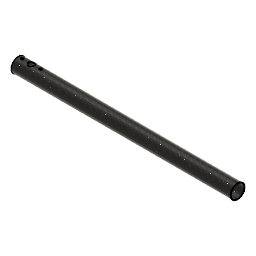
onlydrone (Autodesk Fusion 360 archive; units mm, degrees)
design "Arm"
Autodesk Fusion 360 part; units mm, degrees
sketch "Sketch1" plane through (0, 0, 0) normal (1, 0, 0) x (0, 1, 0)
  circle A0 centre (0, 0) radius 10
  circle A1 centre (0, 0) radius 9
  dimension "d1" = 20
  dimension "d2" = 18
  constraint coincident A0.centre A1.centre
  measures "d1" diameter of A0
  measures "d2" diameter of A1
extrude "Extrude1" add sketch "Sketch1" along normal blind 300
sketch "Sketch2" plane through (0, 0, 0) normal (0, 0, 1) x (1, 0, 0)
  line L0 (0, 0) -> (18, 0) construction
  circle A0 centre (18, 0) radius 4
  line L1 (18, 0) -> (5.5, 0) construction
  circle A1 centre (5.5, 0) radius 1.75
  line L2 (18, 0) -> (18, 4) construction
  line L3 (18, 0) -> (18, 4) construction
  circle A2 centre (30.5, 0) radius 1.75
  dimension "d5" = 18
  dimension "d6" = 8
  dimension "d7" = 12.5
  dimension "d8" = 3.5
  constraint coincident L0.start origin
  constraint horizontal L0
  constraint coincident L0.end A0.centre
  constraint parallel L0 L1
  constraint coincident L1.end A1.centre
  constraint coincident A0 L2.end
  constraint perpendicular L1 L2
  constraint symmetric L0.end L2 A0.centre
  constraint symmetric A1 L2 A2
  constraint symmetric L3.end L2 L2.end
  measures "d5" distance of L0.start L0.end
  measures "d6" diameter of A0
  measures "d7" distance of L0.end L1.end
  measures "d8" diameter of A1
extrude "Extrude2" cut sketch "Sketch2" along normal through all and the other way through all

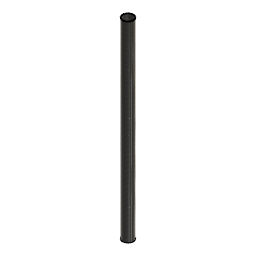
design "Landing Gear"
Autodesk Fusion 360 part; units mm, degrees
sketch "Sketch1" plane through (0, 0, 0) normal (0, 0, 1) x (1, 0, 0)
  circle A0 centre (0, 0) radius 10
  circle A1 centre (0, 0) radius 9
  dimension "d1" = 20
  dimension "d2" = 18
  constraint coincident A0.centre A1.centre
  constraint concentric A0 A1
  measures "d1" diameter of A0
  measures "d2" diameter of A1
extrude "Extrude1" add sketch "Sketch1" along normal blind 250
extrude "Extrude2" add 1 faces at (9.5959, -0.9439, 0) along direction (0, 0, -1) blind 100

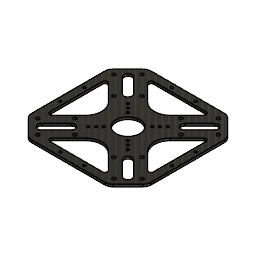
design "Bottom plate"
Autodesk Fusion 360 part; units mm, degrees
sketch "Bottom_Plate" plane through (0, 0, 0) normal (0, 0, 1) x (1, 0, 0)
  line L0 (-65, -33.0086) -> (-65, 33.0086)
  arc A0 (57.6759, 50.6048) -> (50.6048, 57.6759) centre (54.1403, 54.1403) ccw
  line L1 (39.2911, -32.22) -> (57.6759, -50.6048)
  circle A1 centre (0, 0) radius 15
  arc A2 (-33.0086, 65) -> (-35.1299, 59.8787) centre (-33.0086, 62) ccw
  line L2 (46.1091, 75) -> (-46.1091, 75)
  line L3 (57.6759, 50.6048) -> (39.2911, 32.22)
  circle A3 centre (-70, 15) radius 1.5
  circle A4 centre (-15, -70) radius 1.5
  line L4 (-57.6759, -50.6048) -> (-39.2911, -32.22)
  arc A5 (50.6048, -57.6759) -> (57.6759, -50.6048) centre (54.1403, -54.1403) ccw
  circle A6 centre (-15, 70) radius 1.5
  circle A7 centre (-25, -25) radius 1.5
  circle A8 centre (-25, 25) radius 1.5
  circle A9 centre (25, 25) radius 1.5
  circle A10 centre (-42.1195, -24.4419) radius 2
  arc A11 (38.8909, 14.1421) -> (38.8909, -14.1421) centre (53.033, 0) ccw
  circle A12 centre (-15.25, 15.25) radius 1.5
  circle A13 centre (47.7764, -65.4541) radius 2
  line L5 (33.0086, -65) -> (-33.0086, -65)
  arc A14 (-39.2911, 32.22) -> (-32.22, 39.2911) centre (-35.7556, 35.7556) ccw
  arc A15 (32.22, 39.2911) -> (39.2911, 32.22) centre (35.7556, 35.7556) ccw
  line L6 (-32.22, -39.2911) -> (-50.6048, -57.6759)
  arc A16 (-75, -46.1091) -> (-72.0711, -53.1802) centre (-65, -46.1091) ccw
  arc A17 (-32.22, -39.2911) -> (-39.2911, -32.22) centre (-35.7556, -35.7556) ccw
  arc A18 (-57.6759, -50.6048) -> (-50.6048, -57.6759) centre (-54.1403, -54.1403) ccw
  arc A19 (-65, -33.0086) -> (-59.8787, -35.1299) centre (-62, -33.0086) ccw
  arc A20 (59.8787, -35.1299) -> (65, -33.0086) centre (62, -33.0086) ccw
  circle A21 centre (65.4541, -47.7764) radius 2
  line L7 (-14.1421, 38.8909) -> (-35.1299, 59.8787)
  line L8 (72.0711, 53.1802) -> (53.1802, 72.0711)
  line L9 (35.1299, 59.8787) -> (14.1421, 38.8909)
  arc A22 (-59.8787, 35.1299) -> (-65, 33.0086) centre (-62, 33.0086) ccw
  line L10 (59.8787, -35.1299) -> (38.8909, -14.1421)
  arc A23 (35.1299, 59.8787) -> (33.0086, 65) centre (33.0086, 62) ccw
  arc A24 (-53.1802, -72.0711) -> (-46.1091, -75) centre (-46.1091, -65) ccw
  line L11 (38.8909, 14.1421) -> (59.8787, 35.1299)
  circle A25 centre (47.7764, 65.4541) radius 2
  arc A26 (-35.1299, -59.8787) -> (-33.0086, -65) centre (-33.0086, -62) ccw
  line L12 (53.1802, -72.0711) -> (72.0711, -53.1802)
  arc A27 (33.0086, -65) -> (35.1299, -59.8787) centre (33.0086, -62) ccw
  circle A28 centre (-42.1195, 24.4419) radius 2
  circle A29 centre (24.4419, 42.1195) radius 2
  circle A30 centre (15, -70) radius 1.5
  circle A31 centre (-47.7764, 65.4541) radius 2
  line L13 (-33.0086, 65) -> (33.0086, 65)
  arc A32 (-50.6048, 57.6759) -> (-57.6759, 50.6048) centre (-54.1403, 54.1403) ccw
  arc A33 (75, 46.1091) -> (72.0711, 53.1802) centre (65, 46.1091) ccw
  arc A34 (46.1091, -75) -> (53.1802, -72.0711) centre (46.1091, -65) ccw
  line L14 (-53.1802, 72.0711) -> (-72.0711, 53.1802)
  line L15 (-46.1091, -75) -> (46.1091, -75)
  line L16 (-35.1299, -59.8787) -> (-14.1421, -38.8909)
  circle A35 centre (20, -20) radius 1.5
  line L17 (32.22, 39.2911) -> (50.6048, 57.6759)
  circle A36 centre (24.4419, -42.1195) radius 2
  circle A37 centre (20, 20) radius 1.5
  arc A38 (-72.0711, 53.1802) -> (-75, 46.1091) centre (-65, 46.1091) ccw
  arc A39 (39.2911, -32.22) -> (32.22, -39.2911) centre (35.7556, -35.7556) ccw
  arc A40 (72.0711, -53.1802) -> (75, -46.1091) centre (65, -46.1091) ccw
  line L18 (-38.8909, -14.1421) -> (-59.8787, -35.1299)
  circle A41 centre (70, -15) radius 1.5
  line L19 (-59.8787, 35.1299) -> (-38.8909, 14.1421)
  line L20 (-39.2911, 32.22) -> (-57.6759, 50.6048)
  circle A42 centre (15.25, -15.25) radius 1.5
  arc A43 (-38.8909, -14.1421) -> (-38.8909, 14.1421) centre (-53.033, 0) ccw
  line L21 (-72.0711, -53.1802) -> (-53.1802, -72.0711)
  arc A44 (-46.1091, 75) -> (-53.1802, 72.0711) centre (-46.1091, 65) ccw
  line L22 (75, -46.1091) -> (75, 46.1091)
  circle A45 centre (-20, 20) radius 1.5
  circle A46 centre (-70, -15) radius 1.5
  circle A47 centre (-24.4419, -42.1195) radius 2
  arc A48 (53.1802, 72.0711) -> (46.1091, 75) centre (46.1091, 65) ccw
  circle A49 centre (42.1195, -24.4419) radius 2
  arc A50 (-14.1421, 38.8909) -> (14.1421, 38.8909) centre (0, 53.033) ccw
  line L23 (-50.6048, 57.6759) -> (-32.22, 39.2911)
  line L24 (50.6048, -57.6759) -> (32.22, -39.2911)
  circle A51 centre (-24.4419, 42.1195) radius 2
  circle A52 centre (70, 15) radius 1.5
  line L25 (14.1421, -38.8909) -> (35.1299, -59.8787)
  circle A53 centre (-65.4541, -47.7764) radius 2
  circle A54 centre (-15.25, -15.25) radius 1.5
  circle A55 centre (15.25, 15.25) radius 1.5
  arc A56 (65, 33.0086) -> (59.8787, 35.1299) centre (62, 33.0086) ccw
  circle A57 centre (42.1195, 24.4419) radius 2
  line L26 (65, 33.0086) -> (65, -33.0086)
  circle A58 centre (-65.4541, 47.7764) radius 2
  circle A59 centre (65.4541, 47.7764) radius 2
  line L27 (-75, 46.1091) -> (-75, -46.1091)
  arc A60 (14.1421, -38.8909) -> (-14.1421, -38.8909) centre (0, -53.033) ccw
  circle A61 centre (-20, -20) radius 1.5
  circle A62 centre (15, 70) radius 1.5
  circle A63 centre (25, -25) radius 1.5
  circle A64 centre (-47.7764, -65.4541) radius 2
extrude "Extrude1" add sketch "Bottom_Plate" along normal blind 3

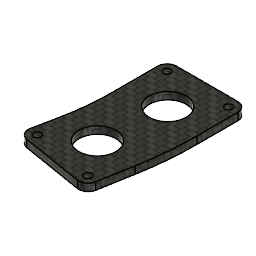
design "Landing Gear plate"
Autodesk Fusion 360 part; units mm, degrees
sketch "Leg_Mount_Plate" plane through (0, 0, 0) normal (0, 0, 1) x (1, 0, 0)
  line L0 (16.25, -4.4078) -> (16.25, 12.25)
  line L1 (11.8234, -41.1043) -> (14.237, -27.4161)
  arc A0 (-20.2099, -35.6287) -> (-17.1464, -40.0699) centre (-16.5339, -36.3702) ccw
  line L2 (-17.1464, -40.0699) -> (7.518, -44.1528)
  arc A1 (-12.5, 16) -> (-16.25, 12.25) centre (-12.5, 12.25) ccw
  arc A2 (14.237, -27.4161) -> (16.25, -4.4078) centre (-116.25, -4.4078) ccw
  line L3 (-16.25, 12.25) -> (-16.25, -6.0136)
  circle A3 centre (-16.5339, -36.3702) radius 1.5
  line L4 (12.5, 16) -> (-12.5, 16)
  circle A4 centre (0, 0) radius 7.5
  circle A5 centre (12.5, 12.25) radius 1.5
  arc A6 (16.25, 12.25) -> (12.5, 16) centre (12.5, 12.25) ccw
  arc A7 (-18.2249, -25.7892) -> (-16.25, -6.0136) centre (-116.25, -6.0136) ccw
  circle A8 centre (8.1304, -40.4531) radius 1.5
  circle A9 centre (-2.2012, -26.3261) radius 7.5
  circle A10 centre (-12.5, 12.25) radius 1.5
  arc A11 (7.518, -44.1528) -> (11.8234, -41.1043) centre (8.1304, -40.4531) ccw
  line L5 (-18.2249, -25.7892) -> (-20.2099, -35.6287)
sketch "Sketch4" plane through (0, 0, 0) normal (0, 0, 1) x (1, 0, 0)
extrude "Extrude1" add sketch "Leg_Mount_Plate" along normal blind 3

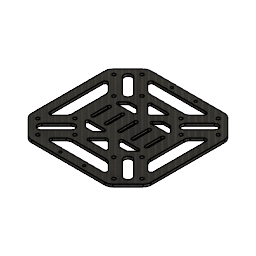
design "Tom Plate"
Autodesk Fusion 360 part; units mm, degrees
sketch "Top_Plate" plane through (0, 0, 0) normal (0, 0, 1) x (1, 0, 0)
  arc A0 (39.2911, -32.22) -> (32.22, -39.2911) centre (35.7556, -35.7556) ccw
  circle A1 centre (24.4419, 42.1195) radius 2
  circle A2 centre (42.1195, -24.4419) radius 2
  circle A3 centre (47.7764, -65.4541) radius 2
  arc A4 (50.6048, -57.6759) -> (57.6759, -50.6048) centre (54.1403, -54.1403) ccw
  circle A5 centre (-47.7764, 65.4541) radius 2
  circle A6 centre (24.4419, -42.1195) radius 2
  arc A7 (51.3431, 26.5944) -> (49, 20.9376) centre (57, 20.9376) ccw
  arc A8 (39.2911, -32.22) -> (32.22, -39.2911) centre (35.7556, -35.7556) ccw
  line L0 (32.22, 39.2911) -> (50.6048, 57.6759)
  line L1 (-57.6759, -50.6048) -> (-39.2911, -32.22)
  circle A9 centre (65.4541, 47.7764) radius 2
  line L2 (-57.6759, -50.6048) -> (-39.2911, -32.22)
  line L3 (-39.2911, 32.22) -> (-57.6759, 50.6048)
  circle A10 centre (-42.1195, 24.4419) radius 2
  line L4 (32.22, 39.2911) -> (50.6048, 57.6759)
  arc A11 (57.6759, 50.6048) -> (50.6048, 57.6759) centre (54.1403, 54.1403) ccw
  circle A12 centre (-24.4419, 42.1195) radius 2
  line L5 (-32.22, -39.2911) -> (-50.6048, -57.6759)
  arc A13 (-32.22, -39.2911) -> (-39.2911, -32.22) centre (-35.7556, -35.7556) ccw
  circle A14 centre (-24.4419, -42.1195) radius 2
  line L6 (59.8787, -35.1299) -> (51.3431, -26.5944)
  circle A15 centre (42.1195, 24.4419) radius 2
  line L7 (51.3431, 26.5944) -> (59.8787, 35.1299)
  line L8 (50.6048, -57.6759) -> (32.22, -39.2911)
  arc A16 (49, -20.9376) -> (51.3431, -26.5944) centre (57, -20.9376) ccw
  arc A17 (-57.6759, -50.6048) -> (-50.6048, -57.6759) centre (-54.1403, -54.1403) ccw
  line L9 (39.2911, -32.22) -> (57.6759, -50.6048)
  line L10 (57.6759, 50.6048) -> (39.2911, 32.22)
  arc A18 (-32.22, -39.2911) -> (-39.2911, -32.22) centre (-35.7556, -35.7556) ccw
  arc A19 (-39.2911, 32.22) -> (-32.22, 39.2911) centre (-35.7556, 35.7556) ccw
  line L11 (57.6759, 50.6048) -> (39.2911, 32.22)
  line L12 (50.6048, -57.6759) -> (32.22, -39.2911)
  arc A20 (-57.6759, -50.6048) -> (-50.6048, -57.6759) centre (-54.1403, -54.1403) ccw
  arc A21 (32.22, 39.2911) -> (39.2911, 32.22) centre (35.7556, 35.7556) ccw
  circle A22 centre (-65.4541, 47.7764) radius 2
  line L13 (-50.6048, 57.6759) -> (-32.22, 39.2911)
  line L14 (-39.2911, 32.22) -> (-57.6759, 50.6048)
  arc A23 (32.22, 39.2911) -> (39.2911, 32.22) centre (35.7556, 35.7556) ccw
  arc A24 (65, 33.0086) -> (59.8787, 35.1299) centre (62, 33.0086) ccw
  arc A25 (-50.6048, 57.6759) -> (-57.6759, 50.6048) centre (-54.1403, 54.1403) ccw
  circle A26 centre (65.4541, -47.7764) radius 2
  arc A27 (32.22, 39.2911) -> (39.2911, 32.22) centre (35.7556, 35.7556) ccw
  arc A28 (50.6048, -57.6759) -> (57.6759, -50.6048) centre (54.1403, -54.1403) ccw
  line L15 (57.6759, 50.6048) -> (39.2911, 32.22)
  circle A29 centre (-24.4419, 42.1195) radius 2
  arc A30 (59.8787, -35.1299) -> (65, -33.0086) centre (62, -33.0086) ccw
  line L16 (-32.22, -39.2911) -> (-50.6048, -57.6759)
  arc A31 (57.6759, 50.6048) -> (50.6048, 57.6759) centre (54.1403, 54.1403) ccw
  arc A32 (-39.2911, 32.22) -> (-32.22, 39.2911) centre (-35.7556, 35.7556) ccw
  line L17 (39.2911, -32.22) -> (57.6759, -50.6048)
  circle A33 centre (-65.4541, -47.7764) radius 2
  line L18 (-33.0086, 65) -> (33.0086, 65)
  circle A34 centre (42.1195, 24.4419) radius 2
  arc A35 (20.9376, 49) -> (26.5944, 51.3431) centre (20.9376, 57) ccw
  arc A36 (-33.0086, 65) -> (-35.1299, 59.8787) centre (-33.0086, 62) ccw
  line L19 (-49, 20.9376) -> (-49, -20.9376)
  line L20 (20.9376, 49) -> (-20.9376, 49)
  arc A37 (50.6048, -57.6759) -> (57.6759, -50.6048) centre (54.1403, -54.1403) ccw
  arc A38 (-26.5944, 51.3431) -> (-20.9376, 49) centre (-20.9376, 57) ccw
  line L21 (-50.6048, 57.6759) -> (-32.22, 39.2911)
  line L22 (50.6048, -57.6759) -> (32.22, -39.2911)
  arc A39 (-20.9376, -49) -> (-26.5944, -51.3431) centre (-20.9376, -57) ccw
  line L23 (65, 33.0086) -> (65, -33.0086)
  arc A40 (-57.6759, -50.6048) -> (-50.6048, -57.6759) centre (-54.1403, -54.1403) ccw
  circle A41 centre (-24.4419, -42.1195) radius 2
  line L24 (49, -20.9376) -> (49, 20.9376)
  line L25 (32.22, 39.2911) -> (50.6048, 57.6759)
  arc A42 (33.0086, -65) -> (35.1299, -59.8787) centre (33.0086, -62) ccw
  circle A43 centre (-42.1195, 24.4419) radius 2
  line L26 (-59.8787, 35.1299) -> (-51.3431, 26.5944)
  arc A44 (51.3431, 26.5944) -> (49, 20.9376) centre (57, 20.9376) ccw
  line L27 (59.8787, -35.1299) -> (51.3431, -26.5944)
  arc A45 (49, -20.9376) -> (51.3431, -26.5944) centre (57, -20.9376) ccw
  circle A46 centre (24.4419, -42.1195) radius 2
  circle A47 centre (-47.7764, 65.4541) radius 2
  circle A48 centre (-65.4541, 47.7764) radius 2
  line L28 (-39.2911, 32.22) -> (-57.6759, 50.6048)
  circle A49 centre (-47.7764, -65.4541) radius 2
  circle A50 centre (65.4541, -47.7764) radius 2
  arc A51 (-50.6048, 57.6759) -> (-57.6759, 50.6048) centre (-54.1403, 54.1403) ccw
  line L29 (33.0086, -65) -> (-33.0086, -65)
  circle A52 centre (47.7764, -65.4541) radius 2
  arc A53 (26.5944, -51.3431) -> (20.9376, -49) centre (20.9376, -57) ccw
  arc A54 (-65, -33.0086) -> (-59.8787, -35.1299) centre (-62, -33.0086) ccw
  arc A55 (32.22, 39.2911) -> (39.2911, 32.22) centre (35.7556, 35.7556) ccw
  circle A56 centre (-47.7764, -65.4541) radius 2
  line L30 (-26.5944, 51.3431) -> (-35.1299, 59.8787)
  line L31 (-20.9376, -49) -> (20.9376, -49)
  arc A57 (39.2911, -32.22) -> (32.22, -39.2911) centre (35.7556, -35.7556) ccw
  line L32 (-65, -33.0086) -> (-65, 33.0086)
  arc A58 (35.1299, 59.8787) -> (33.0086, 65) centre (33.0086, 62) ccw
  arc A59 (-35.1299, -59.8787) -> (-33.0086, -65) centre (-33.0086, -62) ccw
  circle A60 centre (-42.1195, -24.4419) radius 2
  line L33 (39.2911, -32.22) -> (57.6759, -50.6048)
  line L34 (-35.1299, -59.8787) -> (-26.5944, -51.3431)
  circle A61 centre (47.7764, 65.4541) radius 2
  arc A62 (-2, -10) -> (2, -10) centre (0, -10) ccw
  line L35 (-32.22, -39.2911) -> (-50.6048, -57.6759)
  arc A63 (2, 10) -> (-2, 10) centre (0, 10) ccw
  circle A64 centre (65.4541, 47.7764) radius 2
  arc A65 (59.8787, -35.1299) -> (65, -33.0086) centre (62, -33.0086) ccw
  line L36 (2, 10) -> (2, -10)
  line L37 (49, -20.9376) -> (49, 20.9376)
  line L38 (57.6759, 50.6048) -> (39.2911, 32.22)
  arc A66 (57.6759, 50.6048) -> (50.6048, 57.6759) centre (54.1403, 54.1403) ccw
  line L39 (26.5944, -51.3431) -> (35.1299, -59.8787)
  arc A67 (-49, 20.9376) -> (-51.3431, 26.5944) centre (-57, 20.9376) ccw
  circle A68 centre (-65.4541, -47.7764) radius 2
  line L40 (65, 33.0086) -> (65, -33.0086)
  arc A69 (-39.2911, 32.22) -> (-32.22, 39.2911) centre (-35.7556, 35.7556) ccw
  arc A70 (-50.6048, 57.6759) -> (-57.6759, 50.6048) centre (-54.1403, 54.1403) ccw
  circle A71 centre (-24.4419, 42.1195) radius 2
  arc A72 (-51.3431, -26.5944) -> (-49, -20.9376) centre (-57, -20.9376) ccw
  arc A73 (-32.22, -39.2911) -> (-39.2911, -32.22) centre (-35.7556, -35.7556) ccw
  line L41 (20.9376, 49) -> (-20.9376, 49)
  arc A74 (-14.75, 10) -> (-18.75, 10) centre (-16.75, 10) ccw
  line L42 (-18.75, -10) -> (-18.75, 10)
  line L43 (-65, -33.0086) -> (-65, 33.0086)
  circle A75 centre (-47.7764, 65.4541) radius 2
  circle A76 centre (-42.1195, 24.4419) radius 2
  line L44 (32.22, 39.2911) -> (50.6048, 57.6759)
  line L45 (-50.6048, 57.6759) -> (-32.22, 39.2911)
  line L46 (-14.75, 10) -> (-14.75, -10)
  arc A77 (18.75, 10) -> (14.75, 10) centre (16.75, 10) ccw
  line L47 (-20.9376, -49) -> (20.9376, -49)
  line L48 (18.75, 10) -> (18.75, -10)
  arc A78 (14.75, -10) -> (18.75, -10) centre (16.75, -10) ccw
  line L49 (-59.8787, 35.1299) -> (-51.3431, 26.5944)
  circle A79 centre (42.1195, -24.4419) radius 2
  line L50 (26.5944, -51.3431) -> (35.1299, -59.8787)
  line L51 (-51.3431, -26.5944) -> (-59.8787, -35.1299)
  arc A80 (-35.1299, -59.8787) -> (-33.0086, -65) centre (-33.0086, -62) ccw
  line L52 (50.6048, -57.6759) -> (32.22, -39.2911)
  arc A81 (-59.8787, 35.1299) -> (-65, 33.0086) centre (-62, 33.0086) ccw
  circle A82 centre (47.7764, 65.4541) radius 2
  arc A83 (31.5, -10) -> (35.5, -10) centre (33.5, -10) ccw
  line L53 (51.3431, 26.5944) -> (59.8787, 35.1299)
  arc A84 (51.3431, 26.5944) -> (49, 20.9376) centre (57, 20.9376) ccw
  line L54 (35.1299, 59.8787) -> (26.5944, 51.3431)
  arc A85 (-33.0086, 65) -> (-35.1299, 59.8787) centre (-33.0086, 62) ccw
  circle A86 centre (-42.1195, -24.4419) radius 2
  arc A87 (65, 33.0086) -> (59.8787, 35.1299) centre (62, 33.0086) ccw
  line L55 (14.75, -10) -> (14.75, 10)
  arc A88 (-18.75, -10) -> (-14.75, -10) centre (-16.75, -10) ccw
  line L56 (-57.6759, -50.6048) -> (-39.2911, -32.22)
  arc A89 (2, 10) -> (-2, 10) centre (0, 10) ccw
  arc A90 (33.0086, -65) -> (35.1299, -59.8787) centre (33.0086, -62) ccw
  arc A91 (-20.9376, -49) -> (-26.5944, -51.3431) centre (-20.9376, -57) ccw
  line L57 (51.3431, 26.5944) -> (59.8787, 35.1299)
  arc A92 (9.7929, 20.9142) -> (11.2071, 17.5) centre (11.2071, 19.5) ccw
  line L58 (-2, -10) -> (-2, 10)
  arc A93 (-31.5, 10) -> (-35.5, 10) centre (-33.5, 10) ccw
  arc A94 (26.5944, -51.3431) -> (20.9376, -49) centre (20.9376, -57) ccw
  arc A95 (17.4142, 27.5) -> (15.6464, 26.7678) centre (17.4142, 25) ccw
  arc A96 (20.9376, 49) -> (26.5944, 51.3431) centre (20.9376, 57) ccw
  line L59 (-39.2911, 32.22) -> (-57.6759, 50.6048)
  arc A97 (-49, 20.9376) -> (-51.3431, 26.5944) centre (-57, 20.9376) ccw
  line L60 (2, 10) -> (2, -10)
  arc A98 (50.6048, -57.6759) -> (57.6759, -50.6048) centre (54.1403, -54.1403) ccw
  line L61 (-32.6213, 20.9142) -> (-26.7678, 26.7678)
  line L62 (31.5, -10) -> (31.5, 10)
  arc A99 (57.6759, 50.6048) -> (50.6048, 57.6759) centre (54.1403, 54.1403) ccw
  line L63 (-51.3431, -26.5944) -> (-59.8787, -35.1299)
  circle A100 centre (24.4419, 42.1195) radius 2
  line L64 (57.6759, 50.6048) -> (39.2911, 32.22)
  line L65 (-31.5, 10) -> (-31.5, -10)
  line L66 (15.6464, 26.7678) -> (9.7929, 20.9142)
  line L67 (-32.22, -39.2911) -> (-50.6048, -57.6759)
  line L68 (-2, -10) -> (-2, 10)
  circle A101 centre (-65.4541, 47.7764) radius 2
  line L69 (65, 33.0086) -> (65, -33.0086)
  arc A102 (-32.22, -39.2911) -> (-39.2911, -32.22) centre (-35.7556, -35.7556) ccw
  line L70 (-11.2071, 17.5) -> (-31.2071, 17.5)
  line L71 (32.6213, 20.9142) -> (26.7678, 26.7678)
  arc A103 (-65, -33.0086) -> (-59.8787, -35.1299) centre (-62, -33.0086) ccw
  line L72 (33.0086, -65) -> (-33.0086, -65)
  arc A104 (-32.6213, 20.9142) -> (-31.2071, 17.5) centre (-31.2071, 19.5) ccw
  line L73 (-26.5944, 51.3431) -> (-35.1299, 59.8787)
  arc A105 (-26.5944, 51.3431) -> (-20.9376, 49) centre (-20.9376, 57) ccw
  arc A106 (35.1299, 59.8787) -> (33.0086, 65) centre (33.0086, 62) ccw
  line L74 (-49, 20.9376) -> (-49, -20.9376)
  circle A107 centre (65.4541, -47.7764) radius 2
  circle A108 centre (-42.1195, -24.4419) radius 2
  line L75 (-57.6759, -50.6048) -> (-39.2911, -32.22)
  arc A109 (-57.6759, -50.6048) -> (-50.6048, -57.6759) centre (-54.1403, -54.1403) ccw
  arc A110 (-25, 27.5) -> (-26.7678, 26.7678) centre (-25, 25) ccw
  line L76 (14.75, -10) -> (14.75, 10)
  arc A111 (59.8787, -35.1299) -> (65, -33.0086) centre (62, -33.0086) ccw
  line L77 (35.5, 10) -> (35.5, -10)
  arc A112 (-39.2911, 32.22) -> (-32.22, 39.2911) centre (-35.7556, 35.7556) ccw
  arc A113 (-11.2071, 17.5) -> (-9.7929, 20.9142) centre (-11.2071, 19.5) ccw
  line L78 (39.2911, -32.22) -> (57.6759, -50.6048)
  arc A114 (35.5, 10) -> (31.5, 10) centre (33.5, 10) ccw
  arc A115 (49, -20.9376) -> (51.3431, -26.5944) centre (57, -20.9376) ccw
  line L79 (32.22, 39.2911) -> (50.6048, 57.6759)
  circle A116 centre (42.1195, -24.4419) radius 2
  circle A117 centre (24.4419, 42.1195) radius 2
  arc A118 (-51.3431, -26.5944) -> (-49, -20.9376) centre (-57, -20.9376) ccw
  circle A119 centre (-24.4419, -42.1195) radius 2
  line L80 (-15.6464, 26.7678) -> (-9.7929, 20.9142)
  arc A120 (57.6759, 50.6048) -> (50.6048, 57.6759) centre (54.1403, 54.1403) ccw
  line L81 (32.6213, -20.9142) -> (26.7678, -26.7678)
  arc A121 (65, 33.0086) -> (59.8787, 35.1299) centre (62, 33.0086) ccw
  arc A122 (57.6759, 50.6048) -> (50.6048, 57.6759) centre (54.1403, 54.1403) ccw
  circle A123 centre (42.1195, 24.4419) radius 2
  circle A124 centre (-65.4541, 47.7764) radius 2
  line L82 (-15.6464, 26.7678) -> (-9.7929, 20.9142)
  circle A125 centre (-42.1195, 24.4419) radius 2
  line L83 (59.8787, -35.1299) -> (51.3431, -26.5944)
  line L84 (11.2071, -17.5) -> (31.2071, -17.5)
  arc A126 (26.7678, 26.7678) -> (25, 27.5) centre (25, 25) ccw
  arc A127 (-15.6464, 26.7678) -> (-17.4142, 27.5) centre (-17.4142, 25) ccw
  line L85 (-25, 27.5) -> (-17.4142, 27.5)
  arc A128 (31.2071, 17.5) -> (32.6213, 20.9142) centre (31.2071, 19.5) ccw
  circle A129 centre (47.7764, -65.4541) radius 2
  circle A130 centre (-47.7764, -65.4541) radius 2
  circle A131 centre (47.7764, 65.4541) radius 2
  line L86 (-50.6048, 57.6759) -> (-32.22, 39.2911)
  arc A132 (-59.8787, 35.1299) -> (-65, 33.0086) centre (-62, 33.0086) ccw
  circle A133 centre (-65.4541, -47.7764) radius 2
  arc A134 (-2, -10) -> (2, -10) centre (0, -10) ccw
  circle A135 centre (-24.4419, 42.1195) radius 2
  circle A136 centre (65.4541, 47.7764) radius 2
  line L87 (35.1299, 59.8787) -> (26.5944, 51.3431)
  line L88 (-33.0086, 65) -> (33.0086, 65)
  circle A137 centre (-47.7764, 65.4541) radius 2
  arc A138 (-50.6048, 57.6759) -> (-57.6759, 50.6048) centre (-54.1403, 54.1403) ccw
  line L89 (-9.7929, -20.9142) -> (-15.6464, -26.7678)
  line L90 (9.7929, 20.9142) -> (15.6464, 26.7678)
  arc A139 (15.6464, -26.7678) -> (17.4142, -27.5) centre (17.4142, -25) ccw
  line L91 (-18.75, -10) -> (-18.75, 10)
  arc A140 (32.22, 39.2911) -> (39.2911, 32.22) centre (35.7556, 35.7556) ccw
  line L92 (-35.1299, -59.8787) -> (-26.5944, -51.3431)
  line L93 (26.7678, 26.7678) -> (32.6213, 20.9142)
  arc A141 (-35.5, -10) -> (-31.5, -10) centre (-33.5, -10) ccw
  line L94 (25, -27.5) -> (17.4142, -27.5)
  line L95 (-35.5, -10) -> (-35.5, 10)
  line L96 (49, -20.9376) -> (49, 20.9376)
  circle A142 centre (24.4419, -42.1195) radius 2
  line L97 (25, 27.5) -> (17.4142, 27.5)
  arc A143 (39.2911, -32.22) -> (32.22, -39.2911) centre (35.7556, -35.7556) ccw
  line L98 (11.2071, 17.5) -> (31.2071, 17.5)
  arc A144 (9.7929, 20.9142) -> (11.2071, 17.5) centre (11.2071, 19.5) ccw
  line L99 (-11.2071, 17.5) -> (-31.2071, 17.5)
  arc A145 (11.2071, -17.5) -> (9.7929, -20.9142) centre (11.2071, -19.5) ccw
  line L100 (-32.6213, 20.9142) -> (-26.7678, 26.7678)
  arc A146 (-25, 27.5) -> (-26.7678, 26.7678) centre (-25, 25) ccw
  line L101 (-14.75, 10) -> (-14.75, -10)
  arc A147 (51.3431, 26.5944) -> (49, 20.9376) centre (57, 20.9376) ccw
  line L102 (-20.9376, -49) -> (20.9376, -49)
  line L103 (-31.5, 10) -> (-31.5, -10)
  arc A148 (-26.7678, -26.7678) -> (-25, -27.5) centre (-25, -25) ccw
  arc A149 (-15.6464, 26.7678) -> (-17.4142, 27.5) centre (-17.4142, 25) ccw
  arc A150 (-59.8787, 35.1299) -> (-65, 33.0086) centre (-62, 33.0086) ccw
  arc A151 (-20.9376, -49) -> (-26.5944, -51.3431) centre (-20.9376, -57) ccw
  arc A152 (-50.6048, 57.6759) -> (-57.6759, 50.6048) centre (-54.1403, 54.1403) ccw
  arc A153 (32.6213, -20.9142) -> (31.2071, -17.5) centre (31.2071, -19.5) ccw
  arc A154 (31.5, -10) -> (35.5, -10) centre (33.5, -10) ccw
  line L104 (-2, -10) -> (-2, 10)
  line L105 (35.5, 10) -> (35.5, -10)
  line L106 (59.8787, -35.1299) -> (51.3431, -26.5944)
  arc A155 (-1.7678, 26.5165) -> (1.7678, 26.5165) centre (0, 28.2843) ccw
  arc A156 (-49, 20.9376) -> (-51.3431, 26.5944) centre (-57, 20.9376) ccw
  line L107 (-31.2071, -17.5) -> (-11.2071, -17.5)
  arc A157 (-11.2071, 17.5) -> (-9.7929, 20.9142) centre (-11.2071, 19.5) ccw
  line L108 (-49, 20.9376) -> (-49, -20.9376)
  line L109 (15.6464, -26.7678) -> (9.7929, -20.9142)
  arc A158 (14.75, -10) -> (18.75, -10) centre (16.75, -10) ccw
  arc A159 (-39.2911, 32.22) -> (-32.22, 39.2911) centre (-35.7556, 35.7556) ccw
  line L110 (20.9376, 49) -> (-20.9376, 49)
  arc A160 (-18.75, -10) -> (-14.75, -10) centre (-16.75, -10) ccw
  line L111 (18.75, 10) -> (18.75, -10)
  arc A161 (-9.7929, -20.9142) -> (-11.2071, -17.5) centre (-11.2071, -19.5) ccw
  arc A162 (-17.4142, -27.5) -> (-15.6464, -26.7678) centre (-17.4142, -25) ccw
  line L112 (-33.0086, 65) -> (33.0086, 65)
  line L113 (57.6759, 50.6048) -> (39.2911, 32.22)
  line L114 (26.5944, -51.3431) -> (35.1299, -59.8787)
  line L115 (50.6048, -57.6759) -> (32.22, -39.2911)
  arc A163 (-32.22, -39.2911) -> (-39.2911, -32.22) centre (-35.7556, -35.7556) ccw
  arc A164 (65, 33.0086) -> (59.8787, 35.1299) centre (62, 33.0086) ccw
  line L116 (-26.7678, -26.7678) -> (-32.6213, -20.9142)
  arc A165 (-33.0086, 65) -> (-35.1299, 59.8787) centre (-33.0086, 62) ccw
  line L117 (49, -20.9376) -> (49, 20.9376)
  line L118 (-35.5, -10) -> (-35.5, 10)
  arc A166 (31.2071, 17.5) -> (32.6213, 20.9142) centre (31.2071, 19.5) ccw
  arc A167 (39.2911, -32.22) -> (32.22, -39.2911) centre (35.7556, -35.7556) ccw
  line L119 (17.4142, 27.5) -> (25, 27.5)
  arc A168 (18.75, 10) -> (14.75, 10) centre (16.75, 10) ccw
  line L120 (31.2071, 17.5) -> (11.2071, 17.5)
  line L121 (-57.6759, -50.6048) -> (-39.2911, -32.22)
  arc A169 (26.7678, 26.7678) -> (25, 27.5) centre (25, 25) ccw
  arc A170 (2, 10) -> (-2, 10) centre (0, 10) ccw
  arc A171 (-14.75, 10) -> (-18.75, 10) centre (-16.75, 10) ccw
  arc A172 (-26.5944, 51.3431) -> (-20.9376, 49) centre (-20.9376, 57) ccw
  line L122 (-65, -33.0086) -> (-65, 33.0086)
  arc A173 (-35.1299, -59.8787) -> (-33.0086, -65) centre (-33.0086, -62) ccw
  arc A174 (26.5944, -51.3431) -> (20.9376, -49) centre (20.9376, -57) ccw
  arc A175 (50.6048, -57.6759) -> (57.6759, -50.6048) centre (54.1403, -54.1403) ccw
  arc A176 (-51.3431, -26.5944) -> (-49, -20.9376) centre (-57, -20.9376) ccw
  line L123 (35.1299, 59.8787) -> (26.5944, 51.3431)
  line L124 (-32.22, -39.2911) -> (-50.6048, -57.6759)
  arc A177 (33.0086, -65) -> (35.1299, -59.8787) centre (33.0086, -62) ccw
  line L125 (51.3431, 26.5944) -> (59.8787, 35.1299)
  line L126 (39.2911, -32.22) -> (57.6759, -50.6048)
  line L127 (-17.4142, -27.5) -> (-25, -27.5)
  arc A178 (-32.6213, 20.9142) -> (-31.2071, 17.5) centre (-31.2071, 19.5) ccw
  arc A179 (-2, -10) -> (2, -10) centre (0, -10) ccw
  circle A180 centre (24.4419, -42.1195) radius 2
  line L128 (32.22, 39.2911) -> (50.6048, 57.6759)
  line L129 (2, 10) -> (2, -10)
  line L130 (-51.3431, -26.5944) -> (-59.8787, -35.1299)
  line L131 (-25, 27.5) -> (-17.4142, 27.5)
  line L132 (11.2071, -17.5) -> (31.2071, -17.5)
  line L133 (-65, -33.0086) -> (-65, 33.0086)
  arc A181 (9.7929, 20.9142) -> (11.2071, 17.5) centre (11.2071, 19.5) ccw
  line L134 (31.2071, 17.5) -> (11.2071, 17.5)
  line L135 (-35.5, -10) -> (-35.5, 10)
  line L136 (-10.4228, 40) -> (10.4228, 40)
  circle A182 centre (47.7764, -65.4541) radius 2
  arc A183 (32.22, 39.2911) -> (39.2911, 32.22) centre (35.7556, 35.7556) ccw
  line L137 (-39.2911, 32.22) -> (-57.6759, 50.6048)
  arc A184 (25, -27.5) -> (26.7678, -26.7678) centre (25, -25) ccw
  arc A185 (35.5, 10) -> (31.5, 10) centre (33.5, 10) ccw
  arc A186 (59.8787, -35.1299) -> (65, -33.0086) centre (62, -33.0086) ccw
  circle A187 centre (-65.4541, -47.7764) radius 2
  circle A188 centre (-65.4541, 47.7764) radius 2
  arc A189 (20.9376, 49) -> (26.5944, 51.3431) centre (20.9376, 57) ccw
  arc A190 (-10.4228, 40) -> (-11.837, 36.5858) centre (-10.4228, 38) ccw
  circle A191 centre (-24.4419, -42.1195) radius 2
  line L138 (-50.6048, 57.6759) -> (-32.22, 39.2911)
  arc A192 (-35.5, -10) -> (-31.5, -10) centre (-33.5, -10) ccw
  arc A193 (35.1299, 59.8787) -> (33.0086, 65) centre (33.0086, 62) ccw
  line L139 (-35.1299, -59.8787) -> (-26.5944, -51.3431)
  circle A194 centre (42.1195, 24.4419) radius 2
  circle A195 centre (-47.7764, 65.4541) radius 2
  line L140 (11.837, 36.5858) -> (1.7678, 26.5165)
  circle A196 centre (-42.1195, -24.4419) radius 2
  line L141 (-53.1802, 72.0711) -> (-72.0711, 53.1802)
  line L142 (-46.1091, -75) -> (46.1091, -75)
  arc A197 (46.1091, -75) -> (53.1802, -72.0711) centre (46.1091, -65) ccw
  arc A198 (-65, -33.0086) -> (-59.8787, -35.1299) centre (-62, -33.0086) ccw
  line L143 (-18.75, -10) -> (-18.75, 10)
  arc A199 (31.5, -10) -> (35.5, -10) centre (33.5, -10) ccw
  arc A200 (-14.75, 10) -> (-18.75, 10) centre (-16.75, 10) ccw
  arc A201 (-35.5, -10) -> (-31.5, -10) centre (-33.5, -10) ccw
  circle A202 centre (65.4541, 47.7764) radius 2
  arc A203 (-31.2071, -17.5) -> (-32.6213, -20.9142) centre (-31.2071, -19.5) ccw
  arc A204 (2, 10) -> (-2, 10) centre (0, 10) ccw
  line L144 (11.837, 36.5858) -> (1.7678, 26.5165)
  line L145 (33.0086, -65) -> (-33.0086, -65)
  line L146 (-59.8787, 35.1299) -> (-51.3431, 26.5944)
  arc A205 (17.4142, 27.5) -> (15.6464, 26.7678) centre (17.4142, 25) ccw
  circle A206 centre (-24.4419, 42.1195) radius 2
  arc A207 (-10.4228, 40) -> (-11.837, 36.5858) centre (-10.4228, 38) ccw
  circle A208 centre (-42.1195, 24.4419) radius 2
  arc A209 (49, -20.9376) -> (51.3431, -26.5944) centre (57, -20.9376) ccw
  line L147 (31.5, -10) -> (31.5, 10)
  arc A210 (-57.6759, -50.6048) -> (-50.6048, -57.6759) centre (-54.1403, -54.1403) ccw
  line L148 (65, 33.0086) -> (65, -33.0086)
  circle A211 centre (-47.7764, -65.4541) radius 2
  line L149 (-26.5944, 51.3431) -> (-35.1299, 59.8787)
  circle A212 centre (24.4419, 42.1195) radius 2
  line L150 (-11.837, -36.5858) -> (-1.7678, -26.5165)
  arc A213 (-72.0711, 53.1802) -> (-75, 46.1091) centre (-65, 46.1091) ccw
  arc A214 (11.837, 36.5858) -> (10.4228, 40) centre (10.4228, 38) ccw
  circle A215 centre (65.4541, -47.7764) radius 2
  circle A216 centre (47.7764, 65.4541) radius 2
  arc A217 (-31.5, 10) -> (-35.5, 10) centre (-33.5, 10) ccw
  circle A218 centre (42.1195, -24.4419) radius 2
  line L151 (-1.7678, 26.5165) -> (-11.837, 36.5858)
  arc A219 (75, 46.1091) -> (72.0711, 53.1802) centre (65, 46.1091) ccw
  line L152 (2, 10) -> (2, -10)
  line L153 (32.22, 39.2911) -> (50.6048, 57.6759)
  arc A220 (-50.6048, 57.6759) -> (-57.6759, 50.6048) centre (-54.1403, 54.1403) ccw
  line L154 (-31.2071, -17.5) -> (-11.2071, -17.5)
  line L155 (53.1802, -72.0711) -> (72.0711, -53.1802)
  arc A221 (10.4228, -40) -> (11.837, -36.5858) centre (10.4228, -38) ccw
  arc A222 (-1.7678, 26.5165) -> (1.7678, 26.5165) centre (0, 28.2843) ccw
  arc A223 (26.5944, -51.3431) -> (20.9376, -49) centre (20.9376, -57) ccw
  arc A224 (-65, -33.0086) -> (-59.8787, -35.1299) centre (-62, -33.0086) ccw
  line L156 (10.4228, -40) -> (-10.4228, -40)
  arc A225 (53.1802, 72.0711) -> (46.1091, 75) centre (46.1091, 65) ccw
  line L157 (75, -46.1091) -> (75, 46.1091)
  line L158 (-35.1299, -59.8787) -> (-26.5944, -51.3431)
  arc A226 (-26.7678, -26.7678) -> (-25, -27.5) centre (-25, -25) ccw
  arc A227 (-31.2071, -17.5) -> (-32.6213, -20.9142) centre (-31.2071, -19.5) ccw
  line L159 (9.7929, 20.9142) -> (15.6464, 26.7678)
  line L160 (-2, -10) -> (-2, 10)
  arc A228 (-9.7929, -20.9142) -> (-11.2071, -17.5) centre (-11.2071, -19.5) ccw
  arc A229 (-46.1091, 75) -> (-53.1802, 72.0711) centre (-46.1091, 65) ccw
  arc A230 (72.0711, -53.1802) -> (75, -46.1091) centre (65, -46.1091) ccw
  line L161 (-1.7678, 26.5165) -> (-11.837, 36.5858)
  arc A231 (-35.1299, -59.8787) -> (-33.0086, -65) centre (-33.0086, -62) ccw
  line L162 (-75, 46.1091) -> (-75, -46.1091)
  line L163 (35.5, 10) -> (35.5, -10)
  line L164 (25, -27.5) -> (17.4142, -27.5)
  arc A232 (-11.837, -36.5858) -> (-10.4228, -40) centre (-10.4228, -38) ccw
  line L165 (26.5944, -51.3431) -> (35.1299, -59.8787)
  line L166 (20.9376, 49) -> (-20.9376, 49)
  line L167 (15.6464, -26.7678) -> (9.7929, -20.9142)
  line L168 (-14.75, 10) -> (-14.75, -10)
  arc A233 (26.7678, 26.7678) -> (25, 27.5) centre (25, 25) ccw
  line L169 (32.6213, -20.9142) -> (26.7678, -26.7678)
  line L170 (-31.5, 10) -> (-31.5, -10)
  arc A234 (31.2071, 17.5) -> (32.6213, 20.9142) centre (31.2071, 19.5) ccw
  line L171 (-32.6213, 20.9142) -> (-26.7678, 26.7678)
  arc A235 (-51.3431, -26.5944) -> (-49, -20.9376) centre (-57, -20.9376) ccw
  line L172 (72.0711, 53.1802) -> (53.1802, 72.0711)
  line L173 (-26.5944, 51.3431) -> (-35.1299, 59.8787)
  line L174 (31.5, -10) -> (31.5, 10)
  line L175 (-11.2071, 17.5) -> (-31.2071, 17.5)
  arc A236 (1.7678, -26.5165) -> (-1.7678, -26.5165) centre (0, -28.2843) ccw
  line L176 (-15.6464, 26.7678) -> (-9.7929, 20.9142)
  arc A237 (-53.1802, -72.0711) -> (-46.1091, -75) centre (-46.1091, -65) ccw
  line L177 (46.1091, 75) -> (-46.1091, 75)
  arc A238 (15.6464, -26.7678) -> (17.4142, -27.5) centre (17.4142, -25) ccw
  line L178 (-10.4228, 40) -> (10.4228, 40)
  arc A239 (11.2071, -17.5) -> (9.7929, -20.9142) centre (11.2071, -19.5) ccw
  line L179 (-17.4142, -27.5) -> (-25, -27.5)
  arc A240 (35.1299, 59.8787) -> (33.0086, 65) centre (33.0086, 62) ccw
  arc A241 (-20.9376, -49) -> (-26.5944, -51.3431) centre (-20.9376, -57) ccw
  line L180 (-25, 27.5) -> (-17.4142, 27.5)
  arc A242 (11.837, 36.5858) -> (10.4228, 40) centre (10.4228, 38) ccw
  arc A243 (-15.6464, 26.7678) -> (-17.4142, 27.5) centre (-17.4142, 25) ccw
  arc A244 (14.75, -10) -> (18.75, -10) centre (16.75, -10) ccw
  line L181 (-72.0711, -53.1802) -> (-53.1802, -72.0711)
  line L182 (-51.3431, -26.5944) -> (-59.8787, -35.1299)
  line L183 (-49, 20.9376) -> (-49, -20.9376)
  arc A245 (-32.6213, 20.9142) -> (-31.2071, 17.5) centre (-31.2071, 19.5) ccw
  arc A246 (-11.2071, 17.5) -> (-9.7929, 20.9142) centre (-11.2071, 19.5) ccw
  line L184 (35.1299, 59.8787) -> (26.5944, 51.3431)
  arc A247 (-75, -46.1091) -> (-72.0711, -53.1802) centre (-65, -46.1091) ccw
  arc A248 (25, -27.5) -> (26.7678, -26.7678) centre (25, -25) ccw
  arc A249 (-17.4142, -27.5) -> (-15.6464, -26.7678) centre (-17.4142, -25) ccw
  line L185 (-20.9376, -49) -> (20.9376, -49)
  line L186 (65, 33.0086) -> (65, -33.0086)
  circle A250 centre (-42.1195, 24.4419) radius 2
  circle A251 centre (-42.1195, -24.4419) radius 2
  arc A252 (-39.2911, 32.22) -> (-32.22, 39.2911) centre (-35.7556, 35.7556) ccw
  arc A253 (-2, -10) -> (2, -10) centre (0, -10) ccw
  arc A254 (57.6759, 50.6048) -> (50.6048, 57.6759) centre (54.1403, 54.1403) ccw
  arc A255 (32.22, 39.2911) -> (39.2911, 32.22) centre (35.7556, 35.7556) ccw
  line L187 (51.3431, 26.5944) -> (59.8787, 35.1299)
  arc A256 (51.3431, 26.5944) -> (49, 20.9376) centre (57, 20.9376) ccw
  arc A257 (50.6048, -57.6759) -> (57.6759, -50.6048) centre (54.1403, -54.1403) ccw
  arc A258 (33.0086, -65) -> (35.1299, -59.8787) centre (33.0086, -62) ccw
  line L188 (-50.6048, 57.6759) -> (-32.22, 39.2911)
  arc A259 (17.4142, 27.5) -> (15.6464, 26.7678) centre (17.4142, 25) ccw
  circle A260 centre (-24.4419, -42.1195) radius 2
  circle A261 centre (42.1195, 24.4419) radius 2
  circle A262 centre (47.7764, 65.4541) radius 2
  line L189 (33.0086, -65) -> (-33.0086, -65)
  circle A263 centre (24.4419, 42.1195) radius 2
  line L190 (59.8787, -35.1299) -> (51.3431, -26.5944)
  line L191 (26.7678, 26.7678) -> (32.6213, 20.9142)
  arc A264 (35.5, 10) -> (31.5, 10) centre (33.5, 10) ccw
  arc A265 (49, -20.9376) -> (51.3431, -26.5944) centre (57, -20.9376) ccw
  arc A266 (-25, 27.5) -> (-26.7678, 26.7678) centre (-25, 25) ccw
  arc A267 (32.6213, -20.9142) -> (31.2071, -17.5) centre (31.2071, -19.5) ccw
  arc A268 (39.2911, -32.22) -> (32.22, -39.2911) centre (35.7556, -35.7556) ccw
  arc A269 (-59.8787, 35.1299) -> (-65, 33.0086) centre (-62, 33.0086) ccw
  arc A270 (-49, 20.9376) -> (-51.3431, 26.5944) centre (-57, 20.9376) ccw
  circle A271 centre (65.4541, 47.7764) radius 2
  line L192 (57.6759, 50.6048) -> (39.2911, 32.22)
  line L193 (18.75, 10) -> (18.75, -10)
  circle A272 centre (24.4419, -42.1195) radius 2
  arc A273 (18.75, 10) -> (14.75, 10) centre (16.75, 10) ccw
  line L194 (-26.7678, -26.7678) -> (-32.6213, -20.9142)
  circle A274 centre (-15, -70) radius 1.5
  line L195 (39.2911, -32.22) -> (57.6759, -50.6048)
  circle A275 centre (-47.7764, 65.4541) radius 2
  arc A276 (59.8787, -35.1299) -> (65, -33.0086) centre (62, -33.0086) ccw
  circle A277 centre (47.7764, -65.4541) radius 2
  line L196 (-59.8787, 35.1299) -> (-51.3431, 26.5944)
  circle A278 centre (-65.4541, 47.7764) radius 2
  arc A279 (-31.5, 10) -> (-35.5, 10) centre (-33.5, 10) ccw
  line L197 (1.7678, -26.5165) -> (11.837, -36.5858)
  line L198 (-33.0086, 65) -> (33.0086, 65)
  line L199 (-57.6759, -50.6048) -> (-39.2911, -32.22)
  arc A280 (-32.22, -39.2911) -> (-39.2911, -32.22) centre (-35.7556, -35.7556) ccw
  arc A281 (-18.75, -10) -> (-14.75, -10) centre (-16.75, -10) ccw
  line L200 (49, -20.9376) -> (49, 20.9376)
  circle A282 centre (15, -70) radius 1.5
  line L201 (-39.2911, 32.22) -> (-57.6759, 50.6048)
  arc A283 (20.9376, 49) -> (26.5944, 51.3431) centre (20.9376, 57) ccw
  arc A284 (-57.6759, -50.6048) -> (-50.6048, -57.6759) centre (-54.1403, -54.1403) ccw
  arc A285 (-33.0086, 65) -> (-35.1299, 59.8787) centre (-33.0086, 62) ccw
  circle A286 centre (-47.7764, -65.4541) radius 2
  circle A287 centre (65.4541, -47.7764) radius 2
  arc A288 (-26.5944, 51.3431) -> (-20.9376, 49) centre (-20.9376, 57) ccw
  line L202 (14.75, -10) -> (14.75, 10)
  arc A289 (65, 33.0086) -> (59.8787, 35.1299) centre (62, 33.0086) ccw
  line L203 (50.6048, -57.6759) -> (32.22, -39.2911)
  circle A290 centre (42.1195, -24.4419) radius 2
  line L204 (-9.7929, -20.9142) -> (-15.6464, -26.7678)
  circle A291 centre (-24.4419, 42.1195) radius 2
  circle A292 centre (-65.4541, -47.7764) radius 2
  line L205 (17.4142, 27.5) -> (25, 27.5)
  line L206 (-32.22, -39.2911) -> (-50.6048, -57.6759)
extrude "Extrude1" add sketch "Top_Plate" along normal blind 3
sketch "Sketch2" plane through (0, 0, 3) normal (0, 0, 1) x (-1, 0, 0)
  circle A0 centre (42.1195, 24.4419) radius 2
  arc A1 (14.75, -10) -> (18.75, -10) centre (16.75, -10) ccw
  line L0 (14.75, -10) -> (14.75, 10)
  arc A2 (18.75, 10) -> (14.75, 10) centre (16.75, 10) ccw
  line L1 (18.75, 10) -> (18.75, -10)
  arc A3 (-9.7929, -20.9142) -> (-11.2071, -17.5) centre (-11.2071, -19.5) ccw
  line L2 (-9.7929, -20.9142) -> (-15.6464, -26.7678)
  arc A4 (-17.4142, -27.5) -> (-15.6464, -26.7678) centre (-17.4142, -25) ccw
  line L3 (-17.4142, -27.5) -> (-25, -27.5)
  arc A5 (-26.7678, -26.7678) -> (-25, -27.5) centre (-25, -25) ccw
  line L4 (-26.7678, -26.7678) -> (-32.6213, -20.9142)
  arc A6 (-31.2071, -17.5) -> (-32.6213, -20.9142) centre (-31.2071, -19.5) ccw
  line L5 (-31.2071, -17.5) -> (-11.2071, -17.5)
  circle A7 centre (-24.4419, 42.1195) radius 2
  circle A8 centre (47.7764, 65.4541) radius 2
  arc A9 (33.0086, -65) -> (35.1299, -59.8787) centre (33.0086, -62) ccw
  line L6 (33.0086, -65) -> (-33.0086, -65)
  arc A10 (-35.1299, -59.8787) -> (-33.0086, -65) centre (-33.0086, -62) ccw
  line L7 (-35.1299, -59.8787) -> (-26.5944, -51.3431)
  arc A11 (-20.9376, -49) -> (-26.5944, -51.3431) centre (-20.9376, -57) ccw
  line L8 (-20.9376, -49) -> (20.9376, -49)
  arc A12 (26.5944, -51.3431) -> (20.9376, -49) centre (20.9376, -57) ccw
  line L9 (26.5944, -51.3431) -> (35.1299, -59.8787)
  circle A13 centre (24.4419, -42.1195) radius 2
  arc A14 (15.6464, -26.7678) -> (17.4142, -27.5) centre (17.4142, -25) ccw
  line L10 (15.6464, -26.7678) -> (9.7929, -20.9142)
  arc A15 (11.2071, -17.5) -> (9.7929, -20.9142) centre (11.2071, -19.5) ccw
  line L11 (11.2071, -17.5) -> (31.2071, -17.5)
  arc A16 (32.6213, -20.9142) -> (31.2071, -17.5) centre (31.2071, -19.5) ccw
  line L12 (32.6213, -20.9142) -> (26.7678, -26.7678)
  arc A17 (25, -27.5) -> (26.7678, -26.7678) centre (25, -25) ccw
  line L13 (25, -27.5) -> (17.4142, -27.5)
  circle A18 centre (-65.4541, -47.7764) radius 2
  arc A19 (57.6759, 50.6048) -> (50.6048, 57.6759) centre (54.1403, 54.1403) ccw
  line L14 (57.6759, 50.6048) -> (39.2911, 32.22)
  arc A20 (32.22, 39.2911) -> (39.2911, 32.22) centre (35.7556, 35.7556) ccw
  line L15 (32.22, 39.2911) -> (50.6048, 57.6759)
  circle A21 centre (15, 70) radius 1.5
  circle A22 centre (42.1195, -24.4419) radius 2
  circle A23 centre (47.7764, -65.4541) radius 2
  arc A24 (-2, -10) -> (2, -10) centre (0, -10) ccw
  line L16 (-2, -10) -> (-2, 10)
  arc A25 (2, 10) -> (-2, 10) centre (0, 10) ccw
  line L17 (2, 10) -> (2, -10)
  circle A26 centre (-24.4419, -42.1195) radius 2
  arc A27 (35.5, 10) -> (31.5, 10) centre (33.5, 10) ccw
  line L18 (35.5, 10) -> (35.5, -10)
  arc A28 (31.5, -10) -> (35.5, -10) centre (33.5, -10) ccw
  line L19 (31.5, -10) -> (31.5, 10)
  circle A29 centre (-65.4541, 47.7764) radius 2
  arc A30 (-25, 27.5) -> (-26.7678, 26.7678) centre (-25, 25) ccw
  line L20 (-25, 27.5) -> (-17.4142, 27.5)
  arc A31 (-15.6464, 26.7678) -> (-17.4142, 27.5) centre (-17.4142, 25) ccw
  line L21 (-15.6464, 26.7678) -> (-9.7929, 20.9142)
  arc A32 (-11.2071, 17.5) -> (-9.7929, 20.9142) centre (-11.2071, 19.5) ccw
  line L22 (-11.2071, 17.5) -> (-31.2071, 17.5)
  arc A33 (-32.6213, 20.9142) -> (-31.2071, 17.5) centre (-31.2071, 19.5) ccw
  line L23 (-32.6213, 20.9142) -> (-26.7678, 26.7678)
  circle A34 centre (24.4419, 42.1195) radius 2
  circle A35 centre (-47.7764, -65.4541) radius 2
  arc A36 (-31.5, 10) -> (-35.5, 10) centre (-33.5, 10) ccw
  line L24 (-31.5, 10) -> (-31.5, -10)
  arc A37 (-35.5, -10) -> (-31.5, -10) centre (-33.5, -10) ccw
  line L25 (-35.5, -10) -> (-35.5, 10)
  circle A38 centre (-42.1195, -24.4419) radius 2
  arc A39 (75, 46.1091) -> (72.0711, 53.1802) centre (65, 46.1091) ccw
  line L26 (72.0711, 53.1802) -> (53.1802, 72.0711)
  arc A40 (53.1802, 72.0711) -> (46.1091, 75) centre (46.1091, 65) ccw
  line L27 (46.1091, 75) -> (-46.1091, 75)
  arc A41 (-46.1091, 75) -> (-53.1802, 72.0711) centre (-46.1091, 65) ccw
  line L28 (-53.1802, 72.0711) -> (-72.0711, 53.1802)
  arc A42 (-72.0711, 53.1802) -> (-75, 46.1091) centre (-65, 46.1091) ccw
  line L29 (-75, 46.1091) -> (-75, -46.1091)
  arc A43 (-75, -46.1091) -> (-72.0711, -53.1802) centre (-65, -46.1091) ccw
  line L30 (-72.0711, -53.1802) -> (-53.1802, -72.0711)
  arc A44 (-53.1802, -72.0711) -> (-46.1091, -75) centre (-46.1091, -65) ccw
  line L31 (-46.1091, -75) -> (46.1091, -75)
  arc A45 (46.1091, -75) -> (53.1802, -72.0711) centre (46.1091, -65) ccw
  line L32 (53.1802, -72.0711) -> (72.0711, -53.1802)
  arc A46 (72.0711, -53.1802) -> (75, -46.1091) centre (65, -46.1091) ccw
  line L33 (75, -46.1091) -> (75, 46.1091)
  arc A47 (-32.22, -39.2911) -> (-39.2911, -32.22) centre (-35.7556, -35.7556) ccw
  line L34 (-32.22, -39.2911) -> (-50.6048, -57.6759)
  arc A48 (-57.6759, -50.6048) -> (-50.6048, -57.6759) centre (-54.1403, -54.1403) ccw
  line L35 (-57.6759, -50.6048) -> (-39.2911, -32.22)
  circle A49 centre (-15, 70) radius 1.5
  arc A50 (31.2071, 17.5) -> (32.6213, 20.9142) centre (31.2071, 19.5) ccw
  line L36 (31.2071, 17.5) -> (11.2071, 17.5)
  arc A51 (9.7929, 20.9142) -> (11.2071, 17.5) centre (11.2071, 19.5) ccw
  line L37 (9.7929, 20.9142) -> (15.6464, 26.7678)
  arc A52 (17.4142, 27.5) -> (15.6464, 26.7678) centre (17.4142, 25) ccw
  line L38 (17.4142, 27.5) -> (25, 27.5)
  arc A53 (26.7678, 26.7678) -> (25, 27.5) centre (25, 25) ccw
  line L39 (26.7678, 26.7678) -> (32.6213, 20.9142)
  circle A54 centre (65.4541, -47.7764) radius 2
  arc A55 (-26.5944, 51.3431) -> (-20.9376, 49) centre (-20.9376, 57) ccw
  line L40 (-26.5944, 51.3431) -> (-35.1299, 59.8787)
  arc A56 (-33.0086, 65) -> (-35.1299, 59.8787) centre (-33.0086, 62) ccw
  line L41 (-33.0086, 65) -> (33.0086, 65)
  arc A57 (35.1299, 59.8787) -> (33.0086, 65) centre (33.0086, 62) ccw
  line L42 (35.1299, 59.8787) -> (26.5944, 51.3431)
  arc A58 (20.9376, 49) -> (26.5944, 51.3431) centre (20.9376, 57) ccw
  line L43 (20.9376, 49) -> (-20.9376, 49)
  arc A59 (-59.8787, 35.1299) -> (-65, 33.0086) centre (-62, 33.0086) ccw
  line L44 (-59.8787, 35.1299) -> (-51.3431, 26.5944)
  arc A60 (-49, 20.9376) -> (-51.3431, 26.5944) centre (-57, 20.9376) ccw
  line L45 (-49, 20.9376) -> (-49, -20.9376)
  arc A61 (-51.3431, -26.5944) -> (-49, -20.9376) centre (-57, -20.9376) ccw
  line L46 (-51.3431, -26.5944) -> (-59.8787, -35.1299)
  arc A62 (-65, -33.0086) -> (-59.8787, -35.1299) centre (-62, -33.0086) ccw
  line L47 (-65, -33.0086) -> (-65, 33.0086)
  arc A63 (50.6048, -57.6759) -> (57.6759, -50.6048) centre (54.1403, -54.1403) ccw
  line L48 (50.6048, -57.6759) -> (32.22, -39.2911)
  arc A64 (39.2911, -32.22) -> (32.22, -39.2911) centre (35.7556, -35.7556) ccw
  line L49 (39.2911, -32.22) -> (57.6759, -50.6048)
  circle A65 centre (65.4541, 47.7764) radius 2
  arc A66 (1.7678, -26.5165) -> (-1.7678, -26.5165) centre (0, -28.2843) ccw
  line L50 (1.7678, -26.5165) -> (11.837, -36.5858)
  arc A67 (10.4228, -40) -> (11.837, -36.5858) centre (10.4228, -38) ccw
  line L51 (10.4228, -40) -> (-10.4228, -40)
  arc A68 (-11.837, -36.5858) -> (-10.4228, -40) centre (-10.4228, -38) ccw
  line L52 (-11.837, -36.5858) -> (-1.7678, -26.5165)
  arc A69 (-39.2911, 32.22) -> (-32.22, 39.2911) centre (-35.7556, 35.7556) ccw
  line L53 (-39.2911, 32.22) -> (-57.6759, 50.6048)
  arc A70 (-50.6048, 57.6759) -> (-57.6759, 50.6048) centre (-54.1403, 54.1403) ccw
  line L54 (-50.6048, 57.6759) -> (-32.22, 39.2911)
  circle A71 centre (-42.1195, 24.4419) radius 2
  arc A72 (11.837, 36.5858) -> (10.4228, 40) centre (10.4228, 38) ccw
  line L55 (11.837, 36.5858) -> (1.7678, 26.5165)
  arc A73 (-1.7678, 26.5165) -> (1.7678, 26.5165) centre (0, 28.2843) ccw
  line L56 (-1.7678, 26.5165) -> (-11.837, 36.5858)
  arc A74 (-10.4228, 40) -> (-11.837, 36.5858) centre (-10.4228, 38) ccw
  line L57 (-10.4228, 40) -> (10.4228, 40)
  circle A75 centre (-47.7764, 65.4541) radius 2
  arc A76 (-18.75, -10) -> (-14.75, -10) centre (-16.75, -10) ccw
  line L58 (-18.75, -10) -> (-18.75, 10)
  arc A77 (-14.75, 10) -> (-18.75, 10) centre (-16.75, 10) ccw
  line L59 (-14.75, 10) -> (-14.75, -10)
  arc A78 (65, 33.0086) -> (59.8787, 35.1299) centre (62, 33.0086) ccw
  line L60 (65, 33.0086) -> (65, -33.0086)
  arc A79 (59.8787, -35.1299) -> (65, -33.0086) centre (62, -33.0086) ccw
  line L61 (59.8787, -35.1299) -> (51.3431, -26.5944)
  arc A80 (49, -20.9376) -> (51.3431, -26.5944) centre (57, -20.9376) ccw
  line L62 (49, -20.9376) -> (49, 20.9376)
  arc A81 (51.3431, 26.5944) -> (49, 20.9376) centre (57, 20.9376) ccw
  line L63 (51.3431, 26.5944) -> (59.8787, 35.1299)
  line L64 (-75, 0) -> (75, 0) construction
  line L65 (-75, 0) -> (75, 0) construction
  circle A82 centre (15, -70) radius 1.5
  circle A83 centre (-15, -70) radius 1.5
  constraint midpoint L29 L64.start
  constraint midpoint L33 L64.end
  constraint symmetric A21 L64 A82
  constraint symmetric A49 L64 A83
  constraint symmetric L65.start L64 L64.start
  constraint symmetric L65.end L64 L64.end
extrude "Extrude2" cut sketch "Sketch2" against normal blind 7 contours A82 | A83
